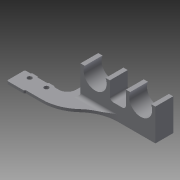
# Autodesk Inventor part: micro-clip
Saved by Autodesk Inventor 2013 (Build 170138000, 138)
## iProperties
Created: 2013-10-16
Part Number: micro-clip
Material: Generic
Document SubType Name: Modeling
Designer: Admin
Density: 1 g/cm^3
Author: Admin
Autodesk Inventor part; units mm, degrees
ref_plane "YZ Plane" through (0, 0, 0) normal (1, 0, 0) x (0, 1, 0)
ref_plane "XZ Plane" through (0, 0, 0) normal (0, 1, 0) x (-1, 0, 0)
ref_plane "XY Plane" through (0, 0, 0) normal (0, 0, 1) x (1, 0, 0)
sketch "Sketch1" plane through (0, 0, 0) normal (0, 0, 1) x (1, 0, 0)
  line L0 (-18.625, 7.0726) -> (-21, 7.0726) projected
  arc A0 (-18.625, 7.0726) -> (-6.875, 7.0726) centre (-12.75, 4.4105) ccw projected
  line L1 (-4.5, 7.0726) -> (-6.875, 7.0726) projected
  line L2 (-4.5, -0.6736) -> (-4.5, 7.0726) projected
  arc A1 (-4.5, -0.6736) -> (-2.5, -2.6736) centre (-2.5, -0.6736) ccw projected
  line L3 (2.5, -2.6736) -> (-2.5, -2.6736) projected
  arc A2 (2.5, -2.6736) -> (4.5, -0.6736) centre (2.5, -0.6736) ccw projected
  line L4 (4.5, 7.0726) -> (4.5, -0.6736) projected
  line L5 (6.875, 7.0726) -> (4.5, 7.0726) projected
  arc A3 (6.875, 7.0726) -> (18.625, 7.0726) centre (12.75, 4.4105) ccw projected
  line L6 (21, 7.0726) -> (18.625, 7.0726) projected
  line L7 (21, 7.0726) -> (21, -6.6736) projected
  line L8 (21, -6.6736) -> (-21, -6.6736) projected
  line L9 (-21, -0.6736) -> (-21, -6.6736) projected
  line L10 (-21, 7.0726) -> (-21, -0.6736) projected
  point P0 (0, 0)
extrude "Extrusion1" add sketch "Sketch1" along normal blind 10
sketch "Sketch2" plane through (-21, -6.6736, 0) normal (0, -1, 0) x (1, 0, 0)
  line L0 (0, 0) -> (42, 0) projected
  line L1 (42, 0) -> (42, 10) projected
  line L2 (0, 10) -> (42, 10) projected
  line L3 (0, 0) -> (0, 10) projected
  line L4 (-19.2077, 22.6478) -> (-27.9377, 22.6478) projected
  arc A0 (-27.9377, 22.6478) -> (-28.6377, 21.9478) centre (-27.9377, 21.9478) ccw projected
  line L5 (-28.6377, 21.9478) -> (-28.6377, 13.1978) projected
  arc A1 (-28.6377, 13.1978) -> (-27.9377, 12.4978) centre (-27.9377, 13.1978) ccw projected
  line L6 (-27.9377, 12.4978) -> (-25.6377, 12.4978) projected
  line L7 (-25.6377, 12.4978) -> (-24.9427, 11.9678) projected
  line L8 (-24.9427, 11.9678) -> (-22.1127, 11.9678) projected
  line L9 (-22.1127, 11.9678) -> (-21.4177, 12.4978) projected
  line L10 (-21.4177, 12.4978) -> (-16.2277, 12.4978) projected
  line L11 (-16.2277, 12.4978) -> (-15.5327, 11.9678) projected
  line L12 (-15.5327, 11.9678) -> (-12.7027, 11.9678) projected
  line L13 (-12.7027, 11.9678) -> (-12.0077, 12.4978) projected
  line L14 (-12.0077, 12.4978) -> (-9.5777, 12.4978) projected
  arc A2 (-9.5777, 12.4978) -> (-8.8777, 13.1978) centre (-9.5777, 13.1978) ccw projected
  line L15 (-8.8777, 13.1978) -> (-8.8777, 21.2678) projected
  arc A3 (-8.8777, 21.2678) -> (-9.5777, 21.9678) centre (-9.5777, 21.2678) ccw projected
  line L16 (-9.5777, 21.9678) -> (-18.5877, 21.9678) projected
  line L17 (-18.5877, 21.9678) -> (-19.2077, 22.6478) projected
  circle A4 centre (-14.1177, 14.9378) radius 1.25 projected
  circle A5 centre (-23.5277, 14.9378) radius 1.25 projected
  arc A6 (5.7111, 15.9839) -> (-9.5777, 21.9678) centre (-9.5777, -0.5556) ccw
  arc A7 (5.7111, 15.9839) -> (21, 10) centre (21, 32.5234) ccw
  arc A8 (-4.7889, 4.7889) -> (0, 0) centre (0, 4.7889) ccw
  line L18 (0, 4.7889) -> (-4.7889, 4.7889) construction
  line L19 (0, 4.7889) -> (0, 0) construction
  arc A9 (-4.7889, 7.709) -> (-9.5777, 12.4978) centre (-9.5777, 7.709) ccw
  line L20 (-9.5777, 7.709) -> (-4.7889, 7.709) construction
  line L21 (-9.5777, 7.709) -> (-9.5777, 12.4978) construction
  line L22 (-4.7889, 7.709) -> (-4.7889, 4.7889)
  point P0 (21, 0)
  dimension "d4" = 90
  dimension "d5" = 90
  constraints: 10 end point, 8 point on circle, 4 centre point, 4 tangent, 2 equal radius, 1 midpoint, 1 parallel, 1 point on line
  measures "d4" angle of L18 L19
  measures "d5" angle of L20 L21
extrude "Extrusion2" add sketch "Sketch2" along normal blind 4.5
sketch "Sketch3" plane through (-21, -6.6736, 0) normal (0, 1, 0) x (1, 0, 0)
  line L0 (0, 0) -> (0, -10) projected
  arc A0 (0, 0) -> (-4.7889, -4.7889) centre (0, -4.7889) ccw projected
  line L1 (-4.7889, -7.709) -> (-4.7889, -4.7889) projected
  arc A1 (-9.5777, -12.4978) -> (-4.7889, -7.709) centre (-9.5777, -7.709) ccw projected
  line L2 (-12.0077, -12.4978) -> (-9.5777, -12.4978) projected
  line L3 (-12.7027, -11.9678) -> (-12.0077, -12.4978) projected
  line L4 (-15.5327, -11.9678) -> (-12.7027, -11.9678) projected
  line L5 (-16.2277, -12.4978) -> (-15.5327, -11.9678) projected
  line L6 (-21.4177, -12.4978) -> (-16.2277, -12.4978) projected
  line L7 (-22.1127, -11.9678) -> (-21.4177, -12.4978) projected
  line L8 (-24.9427, -11.9678) -> (-22.1127, -11.9678) projected
  line L9 (-25.6377, -12.4978) -> (-24.9427, -11.9678) projected
  line L10 (-27.9377, -12.4978) -> (-25.6377, -12.4978) projected
  arc A2 (-27.9377, -12.4978) -> (-28.6377, -13.1978) centre (-27.9377, -13.1978) ccw projected
  line L11 (-28.6377, -21.9478) -> (-28.6377, -13.1978) projected
  arc A3 (-28.6377, -21.9478) -> (-27.9377, -22.6478) centre (-27.9377, -21.9478) ccw projected
  line L12 (-19.2077, -22.6478) -> (-27.9377, -22.6478) projected
  line L13 (-18.5877, -21.9678) -> (-19.2077, -22.6478) projected
  line L14 (-9.5777, -21.9678) -> (-18.5877, -21.9678) projected
  arc A4 (-9.5777, -21.9678) -> (5.7111, -15.9839) centre (-9.5777, 0.5556) ccw projected
  arc A5 (21, -10) -> (5.7111, -15.9839) centre (21, -32.5234) ccw projected
  line L15 (0, -10) -> (21, -10) projected
  circle A6 centre (-23.5277, -14.9378) radius 1.25 projected
  circle A7 centre (-14.1177, -14.9378) radius 1.25 projected
  point P0 (21, 0)
extrude "Extrusion3" cut sketch "Sketch3" against normal blind 2.6259
sketch "Sketch4" plane through (-21, -11.1736, 0) normal (0, -1, 0) x (1, 0, 0)
  circle A0 centre (-23.5277, 14.9378) radius 1.25 projected
  circle A1 centre (-14.1177, 14.9378) radius 1.25 projected
  line L0 (-19.2077, 22.6478) -> (-27.9377, 22.6478) projected
  arc A2 (-27.9377, 22.6478) -> (-28.6377, 21.9478) centre (-27.9377, 21.9478) ccw projected
  line L1 (-28.6377, 21.9478) -> (-28.6377, 13.1978) projected
  arc A3 (-28.6377, 13.1978) -> (-27.9377, 12.4978) centre (-27.9377, 13.1978) ccw projected
  line L2 (-27.9377, 12.4978) -> (-25.6377, 12.4978) projected
  line L3 (-25.6377, 12.4978) -> (-24.9427, 11.9678) projected
  line L4 (-24.9427, 11.9678) -> (-22.1127, 11.9678) projected
  line L5 (-22.1127, 11.9678) -> (-21.4177, 12.4978) projected
  line L6 (-21.4177, 12.4978) -> (-16.2277, 12.4978) projected
  line L7 (-16.2277, 12.4978) -> (-15.5327, 11.9678) projected
  line L8 (-15.5327, 11.9678) -> (-12.7027, 11.9678) projected
  line L9 (-12.7027, 11.9678) -> (-12.0077, 12.4978) projected
  line L10 (-12.0077, 12.4978) -> (-9.5777, 12.4978) projected
  arc A4 (-4.7889, 7.709) -> (-9.5777, 12.4978) centre (-9.5777, 7.709) ccw projected
  line L11 (-4.7889, 7.709) -> (-4.7889, 4.7889) projected
  arc A5 (-4.7889, 4.7889) -> (0, 0) centre (0, 4.7889) ccw projected
  line L12 (0, 0) -> (42, 0) projected
  line L13 (42, 0) -> (42, 10) projected
  line L14 (42, 10) -> (21, 10) projected
  arc A6 (5.7111, 15.9839) -> (21, 10) centre (21, 32.5234) ccw projected
  arc A7 (5.7111, 15.9839) -> (-9.5777, 21.9678) centre (-9.5777, -0.5556) ccw projected
  line L15 (-9.5777, 21.9678) -> (-18.5877, 21.9678) projected
  line L16 (-18.5877, 21.9678) -> (-19.2077, 22.6478) projected
  point P0 (21, 0)
extrude "Extrusion4" cut sketch "Sketch4" against normal blind 0.3741
move or copy body "Move Body1" bodies to move or copy 1 copy no rotation origin (0, 0, 0) rotation axis (-1, 0, 0) rotation angle -90 translate (0, -0.7995, 10.7995)
fillet "Fillet1" radius 2 2 edges at (-10.5, -10.7995, 1.5) (-21, -5.7995, 1.5)
body "Solid1"
